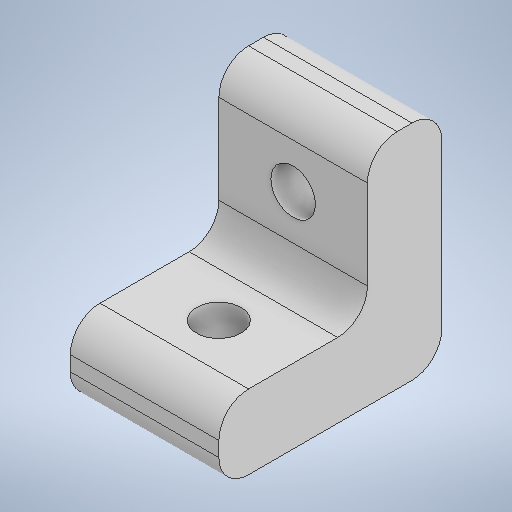
# Autodesk Inventor part: L joint
Saved by Autodesk Inventor 2025.2 (Build 292293000, 293)
## iProperties
Created: 2025-04-09
Part Number: L joint
Material: Generic
Document SubType Name: Modeling
Designer: abdal
Density: 1 g/cm^3
Appearance: Default
Author: abdal
Autodesk Inventor part; units mm, degrees
ref_plane "YZ Plane" through (0, 0, 0) normal (1, 0, 0) x (0, 1, 0)
ref_plane "XZ Plane" through (0, 0, 0) normal (0, 1, 0) x (-1, 0, 0)
ref_plane "XY Plane" through (0, 0, 0) normal (0, 0, 1) x (1, 0, 0)
sketch "Sketch1" plane through (0, 0, 0) normal (1, 0, 0) x (0, 1, 0)
  line L0 (0, 0) -> (5, 0)
  line L1 (5, 5) -> (5, 15)
  line L2 (5, 15) -> (0, 15)
  line L3 (0, 15) -> (0, 0)
  line L4 (0, 0) -> (15, 0)
  line L5 (15, 0) -> (15, 5)
  line L6 (15, 5) -> (5, 5)
  line L7 (0, 15) -> (0, 0)
  point P0 (2.5, 15)
  point P1 (2.5, 0)
  point P2 (0, 7.5)
  point P3 (15, 2.5)
  dimension "d0" = 15
  dimension "d2" = 10
  dimension "d3" = 10
  dimension "d4" = 15
  dimension "d5" = 5
  dimension "d6" = 10
  constraints: 16 end point, 4 midpoint, 4 parallel, 2 horizontal, 2 perpendicular
  measures "d0" distance of point (2.5, 15) point (2.5, 0)
  measures "d2" distance of L1.start L1.end
  measures "d3" distance of L5.end L1.start
  measures "d4" distance between parallel lines of L3 L5
  measures "d5" distance between parallel lines of L0 L6
  measures "d6" distance from line of L7.start L6
extrude "Extrusion1" add sketch "Sketch1" along normal blind 10
fillet "Fillet1" radius 2 6 edges at (5, 5, 5) (5, 0, 0) (5, 5, 15) (5, 0, 15) (5, 15, 5) (5, 15, 0)
sketch "Sketch2" plane through (0, 5, 13) normal (0, 1, 0) x (1, 0, 0)
  circle A0 centre (5, 3) radius 1.5
  line L0 (0, 6) -> (0, 0) projected
  line L1 (0, -2) -> (10, -2) projected
  point P0 (0, 13)
  point P1 (5, -2)
  dimension "d10" = 5
  dimension "d11" = 5
  dimension "d12" = 3
  constraints: 1 centre point, 1 midpoint
  measures "d10" distance from line of L0 A0.centre
  measures "d11" distance of point (5, -2) A0.centre
  measures "d12" diameter of A0
sketch "Sketch3" plane through (0, 7, 5) normal (0, 0, 1) x (1, 0, 0)
  circle A0 centre (5, 3) radius 1.5
  line L0 (10, 8) -> (0, 8) projected
  line L1 (0, 6) -> (0, 0) projected
  point P0 (0, -7)
  point P1 (5, 8)
  point P2 (0, 3)
  dimension "d13" = 3
  dimension "d14" = 5
  dimension "d15" = 5
  constraints: 2 midpoint, 1 centre point
  measures "d13" diameter of A0
  measures "d14" distance of point (5, 8) A0.centre
  measures "d15" distance of point (0, 3) A0.centre
extrude "Extrusion2" cut sketch "Sketch2" against normal through all
extrude "Extrusion3" cut sketch "Sketch3" against normal through all
body "Solid1"
